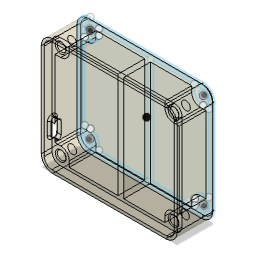
Logger bottom enclosure v34 (Autodesk Fusion 360 design; units mm, degrees)
Autodesk Fusion 360 part; units mm, degrees
note: some values were not read from the file. Set by a fixed rule: which sketch regions a step uses.
sketch "main-bottom" plane through (0, 0, 0) normal (0, 0, 1) x (1, 0, 0)
  line L0 (30, -29) -> (-30, -29)
  line L1 (-34, -25) -> (-34, 25)
  line L2 (-30, 29) -> (30, 29)
  line L3 (34, 25) -> (34, -25)
  arc A0 (-30, 29) -> (-34, 25) centre (-30, 25) ccw
  arc A1 (-34, -25) -> (-30, -29) centre (-30, -25) ccw
  arc A2 (30, -29) -> (34, -25) centre (30, -25) ccw
  arc A3 (34, 25) -> (30, 29) centre (30, 25) ccw
  circle A4 centre (-29.5, 24.5) radius 2.3
  circle A5 centre (29.5, 24.5) radius 2.3
  circle A6 centre (29.5, -24.5) radius 2.3
  circle A7 centre (-29.5, -24.5) radius 2.3
  line L4 (-32.5, -25) -> (-32.5, 25)
  line L5 (32.5, 25) -> (32.5, -25)
  arc A8 (-30, 27.5) -> (-32.5, 25) centre (-30, 25) ccw
  arc A9 (-32.5, -25) -> (-30, -27.5) centre (-30, -25) ccw
  arc A10 (30, -27.5) -> (32.5, -25) centre (30, -25) ccw
  arc A11 (32.5, 25) -> (30, 27.5) centre (30, 25) ccw
  arc A12 (-29.5, 20) -> (-25, 24.5) centre (-29.5, 24.5) ccw
  line L6 (-25, 24.5) -> (-25, 27.5)
  line L7 (-29.5, 20) -> (-32.5, 20)
  line L8 (-29.5, 20) -> (-32.5, 20)
  arc A13 (-29.5, 20) -> (-25, 24.5) centre (-29.5, 24.5) ccw
  line L9 (-25, 24.5) -> (-25, 27.5)
  arc A14 (-29.5, 20) -> (-25, 24.5) centre (-29.5, 24.5) ccw
  line L10 (-25, 24.5) -> (-25, 27.5)
  line L11 (-29.5, 20) -> (-32.5, 20)
  arc A15 (-25, -24.5) -> (-29.5, -20) centre (-29.5, -24.5) ccw
  line L12 (-29.5, -20) -> (-32.5, -20)
  line L13 (-25, -24.5) -> (-25, -27.5)
  arc A16 (29.5, -20) -> (25, -24.5) centre (29.5, -24.5) ccw
  line L14 (25, -24.5) -> (25, -27.5)
  line L15 (29.5, -20) -> (32.5, -20)
  arc A17 (25, 24.5) -> (29.5, 20) centre (29.5, 24.5) ccw
  line L16 (29.5, 20) -> (32.5, 20)
  line L17 (25, 24.5) -> (25, 27.5)
  line L18 (0, -27.5) -> (0.5, -27.5) construction
  line L19 (0, 27.5) -> (0.5, 27.5) construction
  line L20 (0, -27.5) -> (0.5, -27.5)
  line L21 (0, -27.5) -> (0.5, -27.5) construction
  line L22 (3.5, -27.5) -> (3.5, 27.5)
  line L23 (0.5, 27.5) -> (0.5, -27.5)
  line L24 (30, -27.5) -> (3.5, -27.5)
  line L25 (0.5, -27.5) -> (-30, -27.5)
  line L26 (-30, 27.5) -> (0.5, 27.5)
  line L27 (3.5, 27.5) -> (30, 27.5)
  arc A18 (-29.5, 30.5) -> (-35.5, 24.5) centre (-29.5, 24.5) ccw
  line L28 (-29.5, 24.5) -> (-35.5, 24.5) construction
  arc A19 (-29.5, 30.5) -> (-35.5, 24.5) centre (-29.5, 24.5) ccw
  arc A20 (35.5, 24.5) -> (29.5, 30.5) centre (29.5, 24.5) ccw
  arc A21 (-35.5, -24.5) -> (-29.5, -30.5) centre (-29.5, -24.5) ccw
  arc A22 (29.5, -30.5) -> (35.5, -24.5) centre (29.5, -24.5) ccw
  line L29 (-29.5, 30.5) -> (29.5, 30.5)
  line L30 (35.5, 24.5) -> (35.5, -24.5)
  line L31 (29.5, -30.5) -> (-29.5, -30.5)
  line L32 (-35.5, 24.5) -> (-35.5, -24.5)
  dimension "d32" = 4.6
  dimension "d33" = 4.6
  dimension "d34" = 4.6
  dimension "d35" = 4.6
  dimension "d39" = 4.5
  dimension "d40" = 4.5
  dimension "d41" = 4.5
  dimension "d42" = 4.5
  dimension "d43" = 4.5
  dimension "d44" = 4.5
  constraint horizontal L0
  constraint perpendicular L0 L1
  constraint parallel L0 L2
  constraint parallel L1 L3
  constraint tangent L2 A0
  constraint tangent L1 A0
  constraint horizontal L24
  constraint perpendicular L4 L24
  constraint parallel L24 L26
  constraint parallel L4 L5
  constraint coincident A0.centre A8.centre
  constraint coincident A1.centre A9.centre
  constraint coincident A2.centre A10.centre
  constraint coincident A3.centre A11.centre
  constraint coincident A4.centre A12.centre
  constraint coincident L6.end L26
  constraint tangent A12 L6
  constraint perpendicular L6 L26
  constraint coincident L4 L7.end
  constraint tangent A12 L7
  constraint perpendicular L4 L7
  constraint tangent A13 L9
  constraint tangent L8 A13
  constraint tangent A14 L11
  constraint tangent A15 L13
  constraint tangent A16 L15
  constraint tangent A17 L17
  constraint coincident L18.end L24
  constraint parallel L19 L26
  constraint vertical L22
  constraint vertical L23
  constraint collinear L24 L25
  constraint coincident L18.start L24
  constraint collinear L26 L27
  constraint coincident L19.start L26
  constraint tangent A20 L29
  constraint tangent A22 L30
  constraint tangent A21 L31
  constraint tangent A21 L32
  measures "d32" diameter of A4
  measures "d33" diameter of A5
  measures "d34" diameter of A6
  measures "d35" diameter of A7
  measures "d39" radius of A12
  measures "d40" radius of A13
  measures "d41" radius of A14
  measures "d42" radius of A15
  measures "d43" radius of A16
  measures "d44" radius of A17
extrude "Extrude4" add sketch "main-bottom" along normal blind 15.5 contours L0 L1 L2 L3 A0 A1 A2 A3 | A4 | A5 | A6 | A7 | L4 A9 A15 L12 L13 L25 | L4 A8 A12 L6 L7 L8 A13 L9 A14 L10 L11 L26 | L5 A11 A17 L16 L17 L27 | L5 A10 A16 L14 L15 L24 makes body 1
extrude "Extrude3" add sketch "main-bottom" along normal blind 1.5 separate body contours L0 L1 L2 L3 A0 A1 A2 A3 | A4 | A5 | A6 | A7 | L4 A9 A15 L12 L13 L25 | L4 A12 L6 L7 L8 A13 L9 A14 L10 L11 A15 L12 L13 L20 L23 L25 L26 | L4 A8 A12 L6 L7 L8 A13 L9 A14 L10 L11 L26 | L5 A11 A17 L16 L17 L27 | L5 A16 L14 L15 A17 L16 L17 L22 L24 L27 | L5 A10 A16 L14 L15 L24 | A18 A19 A20 A21 A22 L29 L30 L31 L32 makes body 2
extrude "Extrude5" cut sketch "main-bottom" along normal blind 19.6 contours A18 A19 A20 A21 A22 L29 L30 L31 L32 bodies 2
extrude "Extrude6" add sketch "main-bottom" along normal blind 19.6 contours A18 A19 A20 A21 A22 L29 L30 L31 L32 bodies 1 2
hole "Hole1" at (29.5, 24.5, 15.5) direction (0, 0, -1) diameter 4.6 depth 6.5 tip angle 180 countersink diameter 5.6 countersink angle 90 bodies 1
hole "Hole2" at (-29.5, 24.5, 15.5) direction (0, 0, -1) diameter 4.6 depth 6 tip angle 180 countersink diameter 5.6 countersink angle 90 bodies 1
hole "Hole3" at (-29.5, -24.5, 15.5) direction (0, 0, -1) diameter 4.6 depth 6 tip angle 180 countersink diameter 5.6 countersink angle 90 bodies 1
hole "Hole4" at (29.5, -24.5, 15.5) direction (0, 0, -1) diameter 4.6 depth 6 tip angle 180 countersink diameter 5.6 countersink angle 90 bodies 1
sketch "Sketch2" plane through (-35.5, 0, 0) normal (-1, 0, 0) x (0, 0, 1)
  line L0 (0, 24.5) -> (0, -24.5)
  line L1 (0, -24.5) -> (19.6, -24.5)
  line L2 (19.6, -24.5) -> (19.6, 24.5)
  line L3 (19.6, 24.5) -> (0, 24.5)
  line L4 (15.5049, -24.5) -> (15.5049, -19.5) construction
  line L5 (14.1299, -19.5) -> (13.6299, -19.5)
  line L6 (12.2549, -18.125) -> (12.2549, -11.625)
  line L7 (13.6299, -10.25) -> (14.1299, -10.25)
  line L8 (15.5049, -11.625) -> (15.5049, -18.125)
  line L9 (12.2549, -10.25) -> (15.5049, -19.5) construction
  line L10 (12.2549, -19.5) -> (15.5049, -10.25) construction
  line L11 (15.5049, -19.5) -> (14.1299, -19.5) construction
  line L12 (14.1299, -19.5) -> (14.1299, -18.125) construction
  line L13 (14.1299, -18.125) -> (15.5049, -18.125) construction
  line L14 (15.5049, -18.125) -> (15.5049, -19.5) construction
  line L15 (12.2549, -19.5) -> (13.6299, -19.5) construction
  line L16 (13.6299, -19.5) -> (13.6299, -18.125) construction
  line L17 (13.6299, -18.125) -> (12.2549, -18.125) construction
  line L18 (12.2549, -18.125) -> (12.2549, -19.5) construction
  arc A0 (12.2549, -18.125) -> (13.6299, -19.5) centre (13.6299, -18.125) ccw
  arc A1 (15.0049, -18.125) -> (15.004, -18.0743) centre (13.6299, -18.125) ccw
  arc A2 (12.7558, -18.0743) -> (12.7549, -18.125) centre (14.1299, -18.125) ccw
  arc A3 (14.1299, -19.5) -> (15.5049, -18.125) centre (14.1299, -18.125) ccw
  line L19 (15.5049, -10.25) -> (14.1299, -10.25) construction
  line L20 (14.1299, -10.25) -> (14.1299, -11.625) construction
  line L21 (14.1299, -11.625) -> (15.5049, -11.625) construction
  line L22 (15.5049, -11.625) -> (15.5049, -10.25) construction
  line L23 (12.2549, -10.25) -> (13.6299, -10.25) construction
  line L24 (13.6299, -10.25) -> (13.6299, -11.625) construction
  line L25 (13.6299, -11.625) -> (12.2549, -11.625) construction
  line L26 (12.2549, -11.625) -> (12.2549, -10.25) construction
  arc A4 (15.5049, -11.625) -> (14.1299, -10.25) centre (14.1299, -11.625) ccw
  arc A5 (12.7549, -11.625) -> (12.7558, -11.6757) centre (14.1299, -11.625) ccw
  arc A6 (15.004, -11.6757) -> (15.0049, -11.625) centre (13.6299, -11.625) ccw
  arc A7 (13.6299, -10.25) -> (12.2549, -11.625) centre (13.6299, -11.625) ccw
  dimension "d88" = 5
  dimension "d89" = 3.25
  dimension "d90" = 9.25
  dimension "d93" = 1.375
  dimension "d94" = 1.375
  dimension "d95" = 1.375
  dimension "d96" = 1.375
  dimension "d97" = 1.375
  dimension "d98" = 1.375
  dimension "d99" = 1.375
  dimension "d100" = 1.375
  constraint coincident L1 L4.start
  constraint perpendicular L1 L4
  constraint horizontal L5
  constraint vertical L6
  constraint horizontal L7
  constraint vertical L8
  constraint horizontal L11
  constraint vertical L12
  constraint horizontal L13
  constraint vertical L14
  constraint horizontal L15
  constraint vertical L16
  constraint horizontal L17
  constraint vertical L18
  constraint coincident L16.end L17.start
  constraint coincident L12.end L13.start
  constraint coincident L5.start A2
  constraint coincident L13 A1.start
  constraint concentric A0 A1
  constraint coincident L9 A1.end
  constraint coincident L10 A2.start
  constraint coincident L17 A2.end
  constraint concentric A2 A3
  constraint horizontal L19
  constraint vertical L20
  constraint horizontal L21
  constraint vertical L22
  constraint horizontal L23
  constraint vertical L24
  constraint horizontal L25
  constraint vertical L26
  constraint coincident L24.end L25.start
  constraint coincident L7.start A6
  constraint coincident L20.end L21.start
  constraint coincident L10 A6.start
  constraint coincident L9 A5.end
  constraint coincident L25 A5.start
  constraint concentric A4 A5
  constraint coincident L21 A6.end
  constraint concentric A6 A7
  measures "d88" distance of L4.start L4.end
  measures "d89" distance of L4.end L10.start
  measures "d90" distance of L4.end L10.end
  measures "d93" distance of L4.end L5.start
  measures "d94" distance of L4.end L8.end
  measures "d95" distance of L10.start L5.end
  measures "d96" distance of L10.start L6.start
  measures "d97" distance of L10.end L7.end
  measures "d98" distance of L10.end L8.start
  measures "d99" distance of L9.start L7.start
  measures "d100" distance of L9.start L6.end
extrude "Extrude7" cut sketch "Sketch2" against normal blind 3 contours L5 L6 L7 L8 A0 A3 A4 A7 bodies 1
fillet "Fillet1" radius 1 8 edges at (-35.5, -10.25, 13.8799) (-35.5, -10.6527, 15.1022) (-35.5, -14.875, 15.5049) (-35.5, -19.0973, 15.1022) (-35.5, -19.5, 13.8799) (-35.5, -19.0973, 12.6576) (-35.5, -14.875, 12.2549) (-35.5, -10.6527, 12.6576) on bodies 1
fillet "Fillet2" radius 1 8 edges at (33.7426, 28.7426, 0) (0, 30.5, 0) (-33.7426, 28.7426, 0) (-35.5, 0, 0) (-33.7426, -28.7426, 0) (0, -30.5, 0) (33.7426, -28.7426, 0) (35.5, 0, 0) on bodies 1
equation "M3_thread_insert_diameter = 4.6 mm"
equation "d32 = M3_thread_insert_diameter"
equation "d33 = M3_thread_insert_diameter"
equation "d34 = M3_thread_insert_diameter"
equation "d35 = M3_thread_insert_diameter"
equation "bottom_thickness = 1.5 mm"
equation "batholder_height = 13 mm"
equation "batholder_bottom_gap = 1 mm"
equation "FR4_thickness = 1.6 mm"
equation "gasket_thickness = 2.5 mm"
equation "d59 = bottom_thickness"
equation "d61 = bottom_thickness + batholder_bottom_gap + batholder_height"
equation "d63 = bottom_thickness + batholder_bottom_gap + batholder_height + FR4_thickness + gasket_thickness"
equation "d65 = bottom_thickness + batholder_bottom_gap + batholder_height + FR4_thickness + gasket_thickness"
equation "M3_thread_insert_height = 6 mm"
equation "d68 = M3_thread_insert_height + 0.5 mm"
equation "d69 = M3_thread_insert_diameter"
equation "d71 = M3_thread_insert_diameter + 1 mm"
equation "d73 = M3_thread_insert_height"
equation "d74 = M3_thread_insert_diameter"
equation "d76 = M3_thread_insert_diameter + 1 mm"
equation "d78 = M3_thread_insert_height"
equation "d79 = M3_thread_insert_diameter"
equation "d81 = M3_thread_insert_diameter + 1 mm"
equation "d83 = M3_thread_insert_height"
equation "d84 = M3_thread_insert_diameter"
equation "d86 = M3_thread_insert_diameter + 1 mm"
named bodies: "bottom-body"
